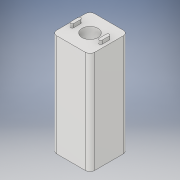
# Autodesk Inventor part: Camera Mount 43mm_all
Saved by Autodesk Inventor 2019 (Build 230136000, 136)
## iProperties
Created: 2020-02-21
Part Number: Camera Mount 43mm_all
Material: Generic
Document SubType Name: Modeling
Designer: close
Density: 1 g/cm^3
Appearance: Smooth - White
Author: close
Autodesk Inventor part; units mm, degrees
ref_plane "YZ Plane" through (0, 0, 0) normal (1, 0, 0) x (0, 1, 0)
ref_plane "XZ Plane" through (0, 0, 0) normal (0, 1, 0) x (-1, 0, 0)
ref_plane "XY Plane" through (0, 0, 0) normal (0, 0, 1) x (1, 0, 0)
sketch "Sketch1" plane through (0, 0, 0) normal (0, 1, 0) x (-1, 0, 0)
  line L0 (6, 8) -> (-6, 8)
  line L1 (-8, 6) -> (-8, -6)
  line L2 (-6, -8) -> (6, -8)
  line L3 (8, -6) -> (8, 6)
  arc A0 (8, 6) -> (6, 8) centre (6, 6) ccw
  arc A1 (-6, 8) -> (-8, 6) centre (-6, 6) ccw
  arc A2 (-8, -6) -> (-6, -8) centre (-6, -6) ccw
  arc A3 (6, -8) -> (8, -6) centre (6, -6) ccw
  point P0 (0, 0)
  point P1 (8, 8)
  point P2 (-8, 8)
  point P3 (8, -8)
  dimension "d0" = 16
  dimension "d1" = 16
  dimension "d2" = 8
  dimension "d3" = 8
  dimension "d4" = 2
  constraints: 8 end point, 8 point on circle, 8 tangent, 6 point on line, 4 centre point, 3 equal radius, 2 parallel, 1 horizontal, 1 perpendicular
  measures "d0" distance of point (8, -8) point (8, 8)
  measures "d1" distance of point (8, 8) point (-8, 8)
  measures "d2" distance from line of L0 point (0, 0)
  measures "d3" distance from line of point (0, 0) L3
  measures "d4" radius of A0
extrude "Extrusion1" add sketch "Sketch1" along normal blind 43
sketch "Sketch2" plane through (0, 0, 0) normal (0, -1, 0) x (1, 0, 0)
  point P0 (0, 0)
hole "Hole1" at (0, 0, 0) direction (0, 1, 0) diameter 6.756 end through all clearance for "Flat Head Machine Screw (82)" size "1/4" standard "Ansi Unified Screw Threads"
sketch "Sketch3" plane through (0, 43, 0) normal (0, 1, 0) x (1, 0, 0)
  line L0 (-6, 1.5) -> (-6, -1.5) construction
  line L1 (-6.65, 1.5) -> (-6.65, -1.5)
  line L2 (-5.35, -1.5) -> (-5.35, 1.5)
  arc A0 (-5.35, 1.5) -> (-6.65, 1.5) centre (-6, 1.5) ccw
  arc A1 (-6.65, -1.5) -> (-5.35, -1.5) centre (-6, -1.5) ccw
  line L3 (6, 1.5) -> (6, -1.5) construction
  line L4 (5.35, 1.5) -> (5.35, -1.5)
  line L5 (6.65, -1.5) -> (6.65, 1.5)
  arc A2 (6.65, 1.5) -> (5.35, 1.5) centre (6, 1.5) ccw
  arc A3 (5.35, -1.5) -> (6.65, -1.5) centre (6, -1.5) ccw
  line L6 (-6, 0) -> (6, 0) construction
  line L7 (6, 8) -> (-6, 8) projected
  point P0 (0, 0)
  dimension "d25" = 0.65
  dimension "d26" = 0.65
  dimension "d27" = 3
  dimension "d29" = 0
  dimension "d30" = 12
  dimension "d31" = 6
  dimension "d32" = 3
  constraints: 18 end point, 8 point on circle, 8 tangent, 4 centre point, 4 parallel, 2 midpoint, 1 vertical
  measures "d25" radius of A0
  measures "d26" radius of A2
  measures "d27" distance of L3.start L3.end
  measures "d29" distance from line of point (0, 0) L6
  measures "d30" distance between parallel lines of L3 L0
  measures "d31" distance of L6.start point (0, 0)
  measures "d32" distance of L0.start L0.end
extrude "Extrusion3" add sketch "Sketch3" along normal blind 1.5
equation "\"d1\" = d0"
equation "\"d2\" = 0.5 * d0"
equation "\"d3\" = d2"
equation "\"d26\" = d25"
equation "\"d27\" = d32"
equation "\"d31\" = 0.5 * d30"
body "Solid1"
